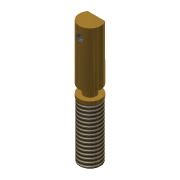
# Autodesk Inventor part: rod
Saved by Autodesk Inventor 2015 (Build 190159000, 159)
## iProperties
Created: 2015-10-28
Part Number: rod
Material: Generic
Document SubType Name: Modeling
Designer: jad211
Density: 1 g/cm^3
Appearance: Default
Author: jad211
Autodesk Inventor part; units mm, degrees
ref_plane "YZ Plane" through (0, 0, 0) normal (1, 0, 0) x (0, 1, 0)
ref_plane "XZ Plane" through (0, 0, 0) normal (0, 1, 0) x (-1, 0, 0)
ref_plane "XY Plane" through (0, 0, 0) normal (0, 0, 1) x (1, 0, 0)
sketch "Sketch1" plane through (0, 0, 0) normal (0, 1, 0) x (-1, 0, 0)
  line L0 (0, 0) -> (-2, 0)
  line L1 (-2, 0) -> (-3.1369, 0)
  line L2 (-3.1369, 0) -> (-3.1369, -16)
  line L3 (-3.1369, -16) -> (-1.7653, -16)
  line L4 (-1.7653, -16) -> (-1.7653, -18.3622)
  line L5 (-1.7653, -18.3622) -> (-3.1369, -18.3622)
  line L6 (-3.1369, -18.3622) -> (-3.1369, -19.3622)
  line L7 (-2, 0) -> (0, 0)
  line L8 (-2, 0) -> (0, 0)
  line L9 (-3.1369, -19.3622) -> (-3, -19.3622)
  line L10 (-3, -19.3622) -> (-3, -35.3622)
  line L11 (-3, -35.3622) -> (0, -35.3622)
  line L12 (0, -35.3622) -> (0, 0)
  dimension "d1" = 0
  dimension "d2" = 16
  dimension "d3" = 2.3622
  dimension "d6" = 3.1369
  dimension "d8" = 3
  dimension "d13" = 1
  dimension "d29" = 1.7653
  dimension "d30" = 16
  constraints: 26 end point, 7 perpendicular, 3 horizontal, 2 point on line, 1 collinear
  measures "d1" distance of L0.end L1.start
  measures "d2" distance of L1.end L2.end
  measures "d3" distance of L3.end L4.end
  measures "d6" distance between parallel lines of L6 L12
  measures "d8" distance of L10.end L11.end
  measures "d13" distance of L5.end L6.end
  measures "d29" distance from line of L12 L3.end
  measures "d30" distance of L9.end L10.end
revolve "Revolution1" add sketch "Sketch1" angle 360 about axis through (0, 0, -35.3622) along (0, 0, 1)
thread "Thread1" size "M6x1" class "6g" standard "ANSI Metric M Profile" full length
sketch "Sketch3" plane through (0, 0, 0) normal (0, 0, 1) x (1, 0, 0)
  circle A0 centre (0, 0) radius 3.1369 projected
  line L0 (-2.4166, -2) -> (2.4166, -2)
  line L1 (-2.5237, 1.8631) -> (2.5237, 1.8631)
  arc A1 (2.4166, -2) -> (2.5237, 1.8631) centre (0, 0) ccw
  arc A2 (-2.5237, 1.8631) -> (-2.4166, -2) centre (0, 0) ccw
  point P0 (0, 0)
  dimension "d36" = 5
  constraints: 8 point on circle, 4 end point, 2 centre point, 1 coincident, 1 horizontal, 1 parallel
extrude "Extrusion1" cut sketch "Sketch3" against normal blind 10 contours L1 A0
sketch "Sketch4" plane through (-2.5237, 1.8631, 0) normal (0, 1, 0) x (1, 0, 0)
  circle A0 centre (2.5237, 3) radius 1
  point P0 (2.5237, 0)
  dimension "d23" = 2
  dimension "d24" = 3
  constraints: 1 centre point
  measures "d23" diameter of A0
  measures "d24" distance of point (2.524, 0) A0.centre
extrude "Extrusion2" cut sketch "Sketch4" against normal blind 10
thread "Thread2" size "M2x0.4" class "6H" standard "ANSI Metric M Profile" full length
sketch "Sketch5" plane through (0, 0, -35.3622) normal (0, 0, -1) x (-1, 0, 0)
  circle A0 centre (0, 0) radius 3.1369 projected
  line L0 (-2.5237, 1.8631) -> (2.5258, 1.8631)
  line L1 (2.5258, 1.8631) -> (2.5258, 4.5959)
  line L2 (2.5258, 4.5959) -> (-2.5237, 4.5959)
  line L3 (-2.5237, 4.5959) -> (-2.5237, 1.8631)
  point P0 (0, 0)
  dimension "d33" = 5
  constraints: 8 end point, 2 parallel, 1 horizontal, 1 perpendicular, 2 other
extrude "Extrusion3" cut sketch "Sketch5" against normal blind 16 contours L0 A0 | A0 L3 L2 L1 picked at (-0.6375, 2.3533)
body "Solid1"
